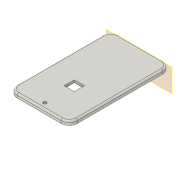
# Autodesk Inventor part: Cover
Saved by Autodesk Inventor 2019 (Build 230136000, 136)
## iProperties
Created: 2019-03-07
Part Number: Cover
Material: PC/ABS Plastic
Document SubType Name: Modeling
Designer: Jared
Density: 0.357273 g/cm^3
Appearance: Steel
Author: Jared
Autodesk Inventor part; units mm, degrees
ref_plane "YZ Plane" through (0, 0, 0) normal (1, 0, 0) x (0, 1, 0)
ref_plane "XZ Plane" through (0, 0, 0) normal (0, 1, 0) x (-1, 0, 0)
ref_plane "XY Plane" through (0, 0, 0) normal (0, 0, 1) x (1, 0, 0)
sketch "Sketch1" plane through (0, 0, 0) normal (0, 1, 0) x (-1, 0, 0)
  line L0 (10, 0) -> (64, 0)
  line L1 (74, -10) -> (74, -115)
  line L2 (64, -125) -> (10, -125)
  line L3 (0, -115) -> (0, -10)
  arc A0 (74, -10) -> (64, 0) centre (64, -10) ccw
  arc A1 (10, 0) -> (0, -10) centre (10, -10) ccw
  arc A2 (0, -115) -> (10, -125) centre (10, -115) ccw
  arc A3 (64, -125) -> (74, -115) centre (64, -115) ccw
  point P0 (0, 0)
  point P1 (74, -125)
  point P2 (0, -125)
  dimension "d0" = 125
  dimension "d1" = 74
  dimension "d2" = 10
  constraints: 8 end point, 8 point on circle, 8 tangent, 6 point on line, 4 centre point, 3 equal radius, 2 parallel, 1 horizontal, 1 perpendicular
  measures "d0" distance between parallel lines of L2 L0
  measures "d1" distance of point (74, -125) point (0, -125)
  measures "d2" radius of A0
extrude "Extrusion1" add sketch "Sketch1" along normal blind 3
sketch "Sketch3" plane through (0, 0, 0) normal (0, -1, 0) x (1, 0, 0)
  line L0 (-64, 0) -> (-10, 0) projected
  arc A0 (-64, 0) -> (-74, -10) centre (-64, -10) ccw projected
  line L1 (-74, -115) -> (-74, -10) projected
  arc A1 (-74, -115) -> (-64, -125) centre (-64, -115) ccw projected
  line L2 (-10, -125) -> (-64, -125) projected
  arc A2 (-10, -125) -> (0, -115) centre (-10, -115) ccw projected
  line L3 (0, -10) -> (0, -115) projected
  arc A3 (0, -10) -> (-10, 0) centre (-10, -10) ccw projected
  line L4 (-10, -2) -> (-64, -2)
  line L5 (-2, -10) -> (-2, -115)
  line L6 (-6.1409, -124.2254) -> (-6.1409, -125)
  line L7 (-72, -115) -> (-72, -10)
  line L8 (-10, -123) -> (-64, -123)
  arc A4 (-2, -10) -> (-10, -2) centre (-10, -10) ccw
  arc A5 (-64, -2) -> (-72, -10) centre (-64, -10) ccw
  arc A6 (-72, -115) -> (-64, -123) centre (-64, -115) ccw
  arc A7 (-10, -123) -> (-2, -115) centre (-10, -115) ccw
  point P0 (0, 0)
  dimension "d5" = 2
  dimension "d6" = 2
  dimension "d7" = 2
  dimension "d8" = 2
  dimension "d10" = 8
  constraints: 10 end point, 9 point on circle, 8 tangent, 4 centre point, 3 equal radius, 3 vertical, 2 horizontal, 1 point on line
  measures "d5" distance between parallel lines of L0 L4
  measures "d6" distance between parallel lines of L3 L5
  measures "d7" distance between parallel lines of L2 L8
  measures "d8" distance between parallel lines of L1 L7
  measures "d10" radius of A4
extrude "Extrusion2" add sketch "Sketch3" along normal blind 2
sketch "Sketch6" plane through (0, 0, 0) normal (0, -1, 0) x (1, 0, 0)
  arc A0 (-2, -10) -> (-10, -2) centre (-10, -10) ccw projected
  line L0 (-10, -2) -> (-64, -2) projected
  arc A1 (-64, -2) -> (-72, -10) centre (-64, -10) ccw projected
  line L1 (-72, -10) -> (-72, -115) projected
  arc A2 (-72, -115) -> (-64, -123) centre (-64, -115) ccw projected
  line L2 (-64, -123) -> (-10, -123) projected
  arc A3 (-10, -123) -> (-2, -115) centre (-10, -115) ccw projected
  line L3 (-2, -115) -> (-2, -10) projected
  line L4 (-43.25, -49.5) -> (-30.75, -49.5)
  line L5 (-30.75, -49.5) -> (-30.75, -37)
  line L6 (-30.75, -37) -> (-43.25, -37)
  line L7 (-43.25, -37) -> (-43.25, -49.5)
  line L8 (-30.75, -43.25) -> (-2, -43.25)
  line L9 (-43.25, -43.25) -> (-72, -43.25)
  line L10 (-72, -115) -> (-72, -10) projected
  point P0 (0, 0)
  dimension "d28" = 12.5
  dimension "d29" = 12.5
  dimension "d41" = 35
  constraints: 12 end point, 3 point on line, 2 horizontal, 2 midpoint, 2 parallel, 1 collinear, 1 perpendicular
  measures "d28" distance of L6.end L5.end
  measures "d29" distance of L5.end L4.end
  measures "d41" distance between parallel lines of L0 L6
extrude "Extrusion4" cut sketch "Sketch6" against normal up to next contours L5 L4 L7 L6
fillet "Fillet1" radius 2 8 edges at (-2.9289, 3, -122.0711) (-37, 3, -125) (-71.0711, 3, -122.0711) (-74, 3, -62.5) (-71.0711, 3, -2.9289) (-37, 3, 0) (-2.9289, 3, -2.9289) (0, 3, -62.5)
ref_plane "Work Plane1" through (-10, 0, -123) normal (0, 0, 1) x (1, 0, 0)
sketch "Sketch8" plane through (-10, 0, -123) normal (0, 0, 1) x (1, 0, 0)
  line L0 (-54, 0) -> (0, 0) projected
  line L1 (-54, 0) -> (-54, -2) projected
  line L2 (0, -2) -> (-54, -2) projected
  line L3 (0, 0) -> (0, -2) projected
  circle A0 centre (-10, -9) radius 4.5
  line L4 (0, -2) -> (-54, -2) projected
  line L5 (-27, -2) -> (-27, -24.2121)
  line L6 (0, 0) -> (0, -2) projected
  line L7 (0, -2) -> (-6.2421, -11.4755)
  line L8 (-13.7579, -11.4755) -> (-20, -2)
  circle A1 centre (-10, -9) radius 1.5
  line L9 (-54, 0) -> (-54, -2)
  circle A2 centre (-44, -9) radius 4.5
  line L10 (-54, 0) -> (-54, -2)
  line L11 (-54, -2) -> (-47.7579, -11.4755)
  line L12 (-40.2421, -11.4755) -> (-34, -2)
  circle A3 centre (-44, -9) radius 1.5
  line L13 (-34, -2) -> (-54, -2)
  point P0 (10, 0)
  dimension "d34" = 7
  dimension "d35" = 9
  dimension "d36" = 10
  dimension "d37" = 10
  dimension "d38" = 3
  constraints: 16 end point, 5 symmetric about line, 4 centre point, 4 point on circle, 2 coincident, 2 tangent, 1 collinear, 1 midpoint, 1 point on line, 1 vertical, 2 other
  measures "d34" distance from line of A0.centre L2
  measures "d35" diameter of A0
  measures "d36" distance from line of L3 A0.centre
  measures "d37" horizontal distance of A0.centre L8.end
  measures "d38" diameter of A1
extrude "Extrusion5" add sketch "Sketch8" along normal blind 2
sketch "Sketch10" plane through (0, 0, 0) normal (0, -1, 0) x (1, 0, 0)
  line L0 (-10, -2) -> (-64, -2) projected
  line L1 (-37, -2) -> (-37, -7)
  circle A0 centre (-37, -7) radius 1.75
  point P0 (0, 0)
  dimension "d42" = 5
  dimension "d43" = 3.5
  constraints: 2 end point, 1 centre point, 1 coincident, 1 midpoint, 1 vertical
  measures "d42" distance of L1.start L1.end
  measures "d43" diameter of A0
extrude "Extrusion6" cut sketch "Sketch10" against normal up to surface (3 mm away)
fillet "Fillet2" radius 0.25 1 edges at (-38.75, 3, -7)
body "Solid1"
